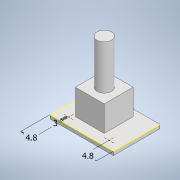
# Autodesk Inventor part: Rotary_Encoder_Model
Saved by Autodesk Inventor 2021 (Build 250183000, 183)
## iProperties
Created: 2020-07-08
Part Number: Rotary_Encoder_Model
Material: Generic
Document SubType Name: Modeling
Designer: ameli
Density: 1 g/cm^3
Appearance: Default
Author: ameli
Autodesk Inventor part; units mm, degrees
ref_plane "YZ Plane" through (0, 0, 0) normal (1, 0, 0) x (0, 1, 0)
ref_plane "XZ Plane" through (0, 0, 0) normal (0, 1, 0) x (-1, 0, 0)
ref_plane "XY Plane" through (0, 0, 0) normal (0, 0, 1) x (1, 0, 0)
sketch "Sketch1" plane through (0, 0, 0) normal (0, 1, 0) x (-1, 0, 0)
  line L0 (13.15, 9.65) -> (-13.15, 9.65)
  line L1 (-13.15, 9.65) -> (-13.15, -9.65)
  line L2 (-13.15, -9.65) -> (13.15, -9.65)
  line L3 (13.15, -9.65) -> (13.15, 9.65)
  point P0 (0, 0)
  dimension "d0" = 19.3
  dimension "d1" = 26.3
  dimension "d2" = 9.65
  dimension "d3" = 13.15
  constraints: 8 end point, 2 parallel, 1 horizontal, 1 perpendicular
  measures "d0" distance of L0.end L1.end
  measures "d1" distance of L1.end L2.end
  measures "d2" distance from line of point (0, 0) L2
  measures "d3" distance from line of point (0, 0) L1
extrude "Extrusion1" add sketch "Sketch1" along normal blind 1.6
sketch "Sketch2" plane through (0, 1.6, 0) normal (0, 1, 0) x (1, 0, 0)
  line L0 (-8.75, -4.25) -> (3.25, -4.25)
  line L1 (3.25, -4.25) -> (3.25, 7.75)
  line L2 (3.25, 7.75) -> (-8.75, 7.75)
  line L3 (-8.75, 7.75) -> (-8.75, -4.25)
  line L4 (13.15, 9.65) -> (-13.15, 9.65) projected
  line L5 (-13.15, 9.65) -> (-13.15, -9.65) projected
  point P0 (0, 0)
  dimension "d6" = 12
  dimension "d7" = 12
  dimension "d8" = 1.9
  dimension "d9" = 4.4
  constraints: 8 end point, 2 parallel, 1 horizontal, 1 perpendicular
  measures "d6" distance of L2.end L0.start
  measures "d7" distance of L1.end L2.end
  measures "d8" distance between parallel lines of L4 L2
  measures "d9" distance between parallel lines of L5 L3
extrude "Extrusion2" add sketch "Sketch2" along normal blind 10.6
sketch "Sketch3" plane through (0, 12.2, 0) normal (0, 1, 0) x (1, 0, 0)
  circle A0 centre (-2.75, 1.75) radius 3
  line L0 (-8.75, 7.75) -> (-8.75, -4.25) projected
  line L1 (3.25, 7.75) -> (-8.75, 7.75) projected
  point P0 (0, 0)
  dimension "d12" = 6
  dimension "d13" = 6
  dimension "d14" = 6
  constraints: 1 centre point
  measures "d12" diameter of A0
  measures "d13" distance from line of L0 A0.centre
  measures "d14" distance from line of L1 A0.centre
extrude "Extrusion3" add sketch "Sketch3" along normal blind 18.4
sketch "Sketch4" plane through (0, 1.6, 0) normal (0, 1, 0) x (1, 0, 0)
  line L0 (-13.15, -9.65) -> (13.15, -9.65) projected
  line L1 (13.15, -9.65) -> (13.15, 9.65) projected
  line L2 (-13.15, 9.65) -> (-13.15, -9.65) projected
  point P0 (0, 0)
  point P1 (-8.35, -6.65)
  point P2 (8.35, -6.65)
  dimension "d17" = 3
  dimension "d18" = 4.8
  dimension "d19" = 4.8
  constraints: 1 horizontal alignment
  measures "d17" distance from line of L0 point (-8.35, -6.65)
  measures "d18" distance from line of L1 point (8.35, -6.65)
  measures "d19" distance from line of L2 point (-8.35, -6.65)
hole "Hole1" at (-8.35, 1.6, 6.65) at (8.35, 1.6, 6.65) direction (0, -1, 0) diameter 2 end through all counterbore diameter 3 counterbore depth 2
body "Solid1"
